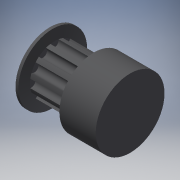
# Autodesk Inventor part: ToothedBeltPulley
Saved by Autodesk Inventor 2018.3 (Build 223284000, 284)
## iProperties
Category: PARTsolutions
Company: MAEDLER
Created: 2018-07-07
Part Number: ToothedBeltPulley
Catalog Web Link: www.cadenas.de
Description: zrr_htd_3m15-HTD Pulleys Profile 3M, Timing Belt Width 15mm
Vendor: MAEDLER
Document SubType Name: Modeling
Designer: psAdmin
Manufacturer: MAEDLER
Mass: 7.4 g
Surface Area: 18.1804 cm^2
Volume: 2.67939 cm^3
Density: 1 g/cm^3
Material: Allgemein
Appearance: PSOLRGB-175-175-175
PSOL_IDENT_0: {$CADENAS_DATA\23d-libs\maedler\antriebselemente\zahnriemenraeder_zahnriemen\zahnriemenraeder\htd-pr
PSOL_IDENT_1: ofil\zrr_htd_3m15.prj},197 {VTYP=3D},{NB=zrr_htd_3m15_0_17031200},{LINA=zrr_htd_3m15_0_17031200},{NN=
PSOL_IDENT_2: zrr_htd_3m15},{DATE=16.06.2017 10:47:49},{GEOMDATE=09.06.2016 09:07:07},{VERSION=},{LINEID=220},{LIN
PSOL_IDENT_3: ESUBID=-1},{WBVAR=BX}  {NB=zrr_htd_3m15_0_17031200},{LINA=zrr_htd_3m15_0_17031200},{KT=DUMMY},{ARTNR=
PSOL_IDENT_4: 17031200},{PDF=PDF Katalogseite},{AUSF=12-3M-15-0F},{MAT=Aluminium},{ZTL=3.000},{ZRB=15.000},{Z=12.0
PSOL_IDENT_5: 00},{AUS=0F},{ZS=10.700},{BS=15.000},{DO=11.460},{ND=15.000},{B=17.000},{L=26.000},{I=0.000},{VB=0.0
PSOL_IDENT_6: 00},{FB=5.000},{BX=0},{GEW=7.400},{ZT=1.200},{ZB=1.800},{T=0.000},{BB=1.000}
NN: zrr_htd_3m15
NT: HTD-Zahnriemenräder Profil 3M, Zahnriemenbreite 15mm
NB: zrr_htd_3m15_0_17031200
NBSYN: zrr_htd_3m15_$BX._$ARTNR.
LINA: zrr_htd_3m15_0_17031200
ARTNR: 17031200
PDF: PDF Katalogseite
AUSF: 12-3M-15-0F
MAT: Aluminium
ZTL: 3.000
ZRB: 15.000
Z: 12.000
AUS: 0F
ZS: 10.700
BS: 15.000
DO: 11.460
ND: 15.000
B: 17.000
L: 26.000
I: 0.000
VB: 0.000
FB: 5.000
BX: 0
GEW: 7.400
ZT: 1.200
ZB: 1.800
T: 0.000
BB: 1.000
SUPPLIER: MAEDLER
ARTICLENO: zrr_htd_3m15_0_17031200
BOMINFO: zrr_htd_3m15_0_17031200
CREATOR: CADENAS GmbH
Title: zrr_htd_3m15_0_17031200
Author: Cadenas PARTsolutions
Comments: HTD Pulleys Profile 3M, Timing Belt Width 15mm
Autodesk Inventor part; units mm, degrees
ref_plane "YZ Plane" through (0, 0, 0) normal (1, 0, 0) x (0, 1, 0)
ref_plane "XZ Plane" through (0, 0, 0) normal (0, 1, 0) x (-1, 0, 0)
ref_plane "XY Plane" through (0, 0, 0) normal (0, 0, 1) x (1, 0, 0)
sketch "Sketch_1" plane through (0, 0, 0) normal (0, 0, 1) x (1, 0, 0)
  line L0 (17.5, 0) -> (0, 0)
  line L1 (0, 0) -> (0, 7.5)
  line L2 (0, 7.5) -> (0.6209, 7.5)
  line L3 (0.6209, 7.5) -> (1, 5.35)
  line L4 (1, 5.35) -> (9.2, 5.35)
  line L5 (9.2, 5.35) -> (9.5791, 7.5)
  line L6 (9.5791, 7.5) -> (10.2, 7.5)
  line L7 (10.2, 7.5) -> (10.2, 7.5)
  line L8 (16.1572, 0) -> (0, 0)
  line L9 (0, 9) -> (0, -1.5) construction
  line L10 (-3.5, 0) -> (21, 0) construction
  line L11 (5.1, 5.35) -> (5.1, 0) construction
  line L12 (10.2, 7.5) -> (17.5, 7.5)
  line L13 (17.5, 7.5) -> (17.5, 0)
  dimension "d3" = 100
  dimension "d4" = 0.6209
  dimension "d5" = 5.35
  dimension "d6" = 7.5
  dimension "d9" = 10.2
  dimension "d10" = 17.5
  dimension "d11" = 7.5
  constraints: 24 end point, 4 collinear, 3 perpendicular, 3 point on line, 2 horizontal, 1 midpoint, 1 other
  measures "d3" angle of L4 L3
  measures "d4" distance of L1.end L2.end
  measures "d5" distance between parallel lines of L10 L4
  measures "d6" distance of L0.end L1.end
  measures "d9" distance between parallel lines of L7 L1
  measures "d10" distance between parallel lines of L13 L1
  measures "d11" distance between parallel lines of L0 L12
revolve "Revolution1" add sketch "Sketch_1" angle 360 about axis through (17.5, 0, 0) along (-1, 0, 0)
sketch "Sketch_2" plane through (1, 0, 0) normal (1, 0, 0) x (0, 0, -1)
  circle A0 centre (0, 0) radius 10.7
  line L0 (-5.2738, 0.9) -> (-5.05, 0.9)
  arc A1 (-4.15, 0) -> (-5.05, 0.9) centre (-5.05, 0) ccw
  arc A2 (-5.05, -0.9) -> (-4.15, 0) centre (-5.05, 0) ccw
  line L1 (-5.05, -0.9) -> (-5.2738, -0.9)
  arc A3 (-5.2738, -0.9) -> (-5.1677, -1.3847) centre (0, 0) ccw
  arc A4 (-5.1677, -1.3847) -> (-5.0172, -1.8575) centre (0, 0) ccw
  line L2 (-5.0172, -1.8575) -> (-4.8234, -1.7456)
  arc A5 (-3.594, -2.075) -> (-4.8234, -1.7456) centre (-4.3734, -2.525) ccw
  arc A6 (-3.9234, -3.3044) -> (-3.594, -2.075) centre (-4.3734, -2.525) ccw
  line L3 (-3.9234, -3.3044) -> (-4.1172, -3.4163)
  arc A7 (-4.1172, -3.4163) -> (-3.783, -3.783) centre (0, 0) ccw
  arc A8 (-3.783, -3.783) -> (-3.4163, -4.1172) centre (0, 0) ccw
  line L4 (-3.4163, -4.1172) -> (-3.3044, -3.9234)
  arc A9 (-2.075, -3.594) -> (-3.3044, -3.9234) centre (-2.525, -4.3734) ccw
  arc A10 (-1.7456, -4.8234) -> (-2.075, -3.594) centre (-2.525, -4.3734) ccw
  line L5 (-1.7456, -4.8234) -> (-1.8575, -5.0172)
  arc A11 (-1.8575, -5.0172) -> (-1.3847, -5.1677) centre (0, 0) ccw
  arc A12 (-1.3847, -5.1677) -> (-0.9, -5.2738) centre (0, 0) ccw
  line L6 (-0.9, -5.2738) -> (-0.9, -5.05)
  arc A13 (0, -4.15) -> (-0.9, -5.05) centre (0, -5.05) ccw
  arc A14 (0.9, -5.05) -> (0, -4.15) centre (0, -5.05) ccw
  line L7 (0.9, -5.05) -> (0.9, -5.2738)
  arc A15 (0.9, -5.2738) -> (1.3847, -5.1677) centre (0, 0) ccw
  arc A16 (1.3847, -5.1677) -> (1.8575, -5.0172) centre (0, 0) ccw
  line L8 (1.8575, -5.0172) -> (1.7456, -4.8234)
  arc A17 (2.075, -3.594) -> (1.7456, -4.8234) centre (2.525, -4.3734) ccw
  arc A18 (3.3044, -3.9234) -> (2.075, -3.594) centre (2.525, -4.3734) ccw
  line L9 (3.3044, -3.9234) -> (3.4163, -4.1172)
  arc A19 (3.4163, -4.1172) -> (3.783, -3.783) centre (0, 0) ccw
  arc A20 (3.783, -3.783) -> (4.1172, -3.4163) centre (0, 0) ccw
  line L10 (4.1172, -3.4163) -> (3.9234, -3.3044)
  arc A21 (3.594, -2.075) -> (3.9234, -3.3044) centre (4.3734, -2.525) ccw
  arc A22 (4.8234, -1.7456) -> (3.594, -2.075) centre (4.3734, -2.525) ccw
  line L11 (4.8234, -1.7456) -> (5.0172, -1.8575)
  arc A23 (5.0172, -1.8575) -> (5.1677, -1.3847) centre (0, 0) ccw
  arc A24 (5.1677, -1.3847) -> (5.2738, -0.9) centre (0, 0) ccw
  line L12 (5.2738, -0.9) -> (5.05, -0.9)
  arc A25 (4.15, 0) -> (5.05, -0.9) centre (5.05, 0) ccw
  arc A26 (5.05, 0.9) -> (4.15, 0) centre (5.05, 0) ccw
  line L13 (5.05, 0.9) -> (5.2738, 0.9)
  arc A27 (5.2738, 0.9) -> (5.1677, 1.3847) centre (0, 0) ccw
  arc A28 (5.1677, 1.3847) -> (5.0172, 1.8575) centre (0, 0) ccw
  line L14 (5.0172, 1.8575) -> (4.8234, 1.7456)
  arc A29 (3.594, 2.075) -> (4.8234, 1.7456) centre (4.3734, 2.525) ccw
  arc A30 (3.9234, 3.3044) -> (3.594, 2.075) centre (4.3734, 2.525) ccw
  line L15 (3.9234, 3.3044) -> (4.1172, 3.4163)
  arc A31 (4.1172, 3.4163) -> (3.783, 3.783) centre (0, 0) ccw
  arc A32 (3.783, 3.783) -> (3.4163, 4.1172) centre (0, 0) ccw
  line L16 (3.4163, 4.1172) -> (3.3044, 3.9234)
  arc A33 (2.075, 3.594) -> (3.3044, 3.9234) centre (2.525, 4.3734) ccw
  arc A34 (1.7456, 4.8234) -> (2.075, 3.594) centre (2.525, 4.3734) ccw
  line L17 (1.7456, 4.8234) -> (1.8575, 5.0172)
  arc A35 (1.8575, 5.0172) -> (1.3847, 5.1677) centre (0, 0) ccw
  arc A36 (1.3847, 5.1677) -> (0.9, 5.2738) centre (0, 0) ccw
  line L18 (0.9, 5.2738) -> (0.9, 5.05)
  arc A37 (0, 4.15) -> (0.9, 5.05) centre (0, 5.05) ccw
  arc A38 (-0.9, 5.05) -> (0, 4.15) centre (0, 5.05) ccw
  line L19 (-0.9, 5.05) -> (-0.9, 5.2738)
  arc A39 (-0.9, 5.2738) -> (-1.3847, 5.1677) centre (0, 0) ccw
  arc A40 (-1.3847, 5.1677) -> (-1.8575, 5.0172) centre (0, 0) ccw
  line L20 (-1.8575, 5.0172) -> (-1.7456, 4.8234)
  arc A41 (-2.075, 3.594) -> (-1.7456, 4.8234) centre (-2.525, 4.3734) ccw
  arc A42 (-3.3044, 3.9234) -> (-2.075, 3.594) centre (-2.525, 4.3734) ccw
  line L21 (-3.3044, 3.9234) -> (-3.4163, 4.1172)
  arc A43 (-3.4163, 4.1172) -> (-3.783, 3.783) centre (0, 0) ccw
  arc A44 (-3.783, 3.783) -> (-4.1172, 3.4163) centre (0, 0) ccw
  line L22 (-4.1172, 3.4163) -> (-3.9234, 3.3044)
  arc A45 (-3.594, 2.075) -> (-3.9234, 3.3044) centre (-4.3734, 2.525) ccw
  arc A46 (-4.8234, 1.7456) -> (-3.594, 2.075) centre (-4.3734, 2.525) ccw
  line L23 (-4.8234, 1.7456) -> (-5.0172, 1.8575)
  arc A47 (-5.0172, 1.8575) -> (-5.1677, 1.3847) centre (0, 0) ccw
  arc A48 (-5.1677, 1.3847) -> (-5.2738, 0.9) centre (0, 0) ccw
  line L24 (0, 0) -> (0, 5.05) construction
  line L25 (0, 0) -> (-2.525, 4.3734) construction
  dimension "d8" = 30
  constraints: 96 point on circle, 52 end point, 49 centre point, 1 vertical
  measures "d8" angle of L25 L24
extrude "Extrusion1" cut sketch "Sketch_2" along normal blind 8
body "Solid1"
